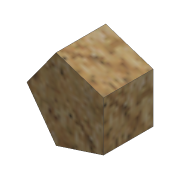
# Autodesk Inventor part: 土壤
Saved by Autodesk Inventor 2018 (Build 220112000, 112)
## iProperties
Created: 2021-03-10
Part Number: 土壤
Material: 常规
Document SubType Name: Modeling
Designer: OHHHHHHHHHH
Density: 1 g/cm^3
Appearance: 刨花板
Author: OHHHHHHHHHH
Autodesk Inventor part; units mm, degrees
ref_plane "YZ Plane" through (0, 0, 0) normal (1, 0, 0) x (0, 1, 0)
ref_plane "XZ Plane" through (0, 0, 0) normal (0, 1, 0) x (-1, 0, 0)
ref_plane "XY Plane" through (0, 0, 0) normal (0, 0, 1) x (1, 0, 0)
sketch "草图1" plane through (0, 0, 0) normal (0, 1, 0) x (-1, 0, 0)
  line L0 (68.3073, 0) -> (21.1081, -64.9641)
  line L1 (21.1081, -64.9641) -> (-55.2617, -40.15)
  line L2 (-55.2617, -40.15) -> (-55.2617, 40.15)
  line L3 (-55.2617, 40.15) -> (21.1081, 64.9641)
  line L4 (21.1081, 64.9641) -> (68.3073, 0)
  point P0 (0, 0)
  point P1 (0, 0)
  point P2 (0, 0)
  point P3 (0, 0)
  dimension "d0" = 80.3
  constraints: 10 end point, 2 coincident, 11 other
  measures "d0" distance of L1.end L2.end
extrude "拉伸1" add sketch "草图1" along normal blind 80
